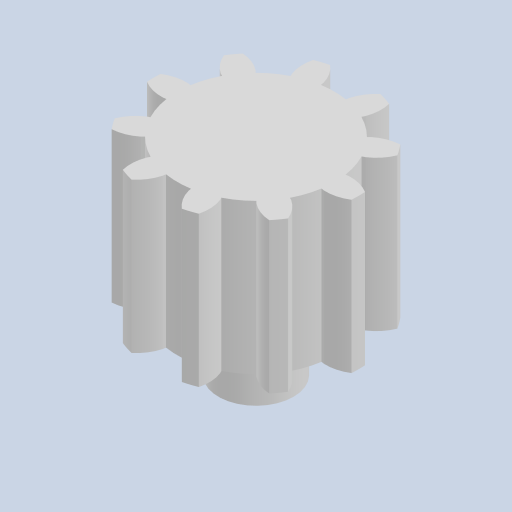
# Autodesk Inventor part: planeta_V2
Saved by Autodesk Inventor 2024 (Build 280153000, 153)
## iProperties
Created: 2023-12-10
Part Number: planeta_V2
Material: Generic
Document SubType Name: Modeling
Designer: mirun
Density: 1 g/cm^3
Appearance: Default
Author: mirun
Autodesk Inventor part; units mm, degrees
ref_plane "YZ Plane" through (0, 0, 0) normal (1, 0, 0) x (0, 1, 0)
ref_plane "XZ Plane" through (0, 0, 0) normal (0, 1, 0) x (-1, 0, 0)
ref_plane "XY Plane" through (0, 0, 0) normal (0, 0, 1) x (1, 0, 0)
sketch "Sketch1" plane through (0, 0, 0) normal (0, 1, 0) x (-1, 0, 0)
  circle A0 centre (0, 0) radius 6.125 construction
  circle A1 centre (0, 0) radius 6.825
  circle A2 centre (0, 0) radius 5.225
  circle A3 centre (0, 0) radius 5.425 construction
  line L0 (0, 0) -> (5.225, 0) construction
  line L1 (6.825, 0) -> (5.1994, 0) construction
  line L2 (6.125, 0) -> (6.825, 0) construction
  line L3 (5.425, 0) -> (6.125, 0) construction
  line L4 (5.225, 0) -> (5.425, 0) construction
  line L5 (5.361, -0.8306) -> (5.1634, -0.8)
  arc A4 (5.361, -0.8306) -> (6.8101, -0.45) centre (5.4797, 1.6666) ccw
  line L6 (5.361, 0.8306) -> (5.1634, 0.8)
  arc A5 (6.8101, 0.45) -> (5.361, 0.8306) centre (5.4797, -1.6666) ccw
  point P0 (5.1634, 0.8)
  point P1 (6.8101, 0.45)
  dimension "d0" = 12.25
  dimension "d1" = 0.7
  dimension "d2" = 0.7
  dimension "d3" = 0.2
  dimension "d4" = 0.8
  dimension "d5" = 2.5
  dimension "d6" = 0.45
  constraints: 14 end point, 10 point on circle, 5 centre point, 5 horizontal, 4 coincident, 4 symmetric about line, 1 horizontal alignment, 1 line through centre, 3 other
  measures "d1" distance of L2.start L1.start
  measures "d2" distance of L3.start L2.start
  measures "d3" distance of L0.end L3.start
  measures "d4" vertical distance of L5.end L0.end
  measures "d5" radius of A4
  measures "d6" vertical distance of L1.start A1.end
extrude "Extrusion1" add sketch "Sketch1" along normal blind 10 contours A1 A4 L5 A2 L6 A5 | A2 picked at (5.9792, 0)
pattern_circular "Circular Pattern1" count 10 over 360 about axis through (0, 0, 0) along (0, 1, 0) of "Extrusion1"
sketch "Sketch3" plane through (0, 0, 0) normal (0, -1, 0) x (1, 0, 0)
  arc A0 (-4.6475, 2.3878) -> (-5.1634, 0.8) centre (0, 0) ccw construction
  circle A1 centre (0, 0) radius 2.5
  dimension "d13" = 5
  constraints: 1 centre point, 1 coincident
  measures "d13" diameter of A1
extrude "Extrusion2" add sketch "Sketch3" along normal blind 3.75
body "Solid1"
